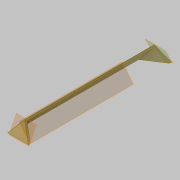
# Autodesk Inventor part: ESTAMP Post 6832 Gold L=149; BC=128
Saved by Autodesk Inventor 2024 (Build 280153000, 153)
## iProperties
Created: 2023-02-20
Part Number: ESTAMP Post 6832 Gold L=149; BC=128
Material: Zinc
Document SubType Name: Modeling
Designer: sauliusd
Density: 7 g/cm^3
Appearance: Gold - Metal
Description: ESTAMP Handle Post 683
Appearance: Chrome - Polished Black
Author: sauliusd
Autodesk Inventor part; units mm, degrees
ref_plane "YZ Plane" through (0, 0, 0) normal (1, 0, 0) x (0, 1, 0)
ref_plane "XZ Plane" through (0, 0, 0) normal (0, 1, 0) x (-1, 0, 0)
ref_plane "XY Plane" through (0, 0, 0) normal (0, 0, 1) x (1, 0, 0)
sketch "Sketch1" plane through (0, 0, 0) normal (0, 0, 1) x (1, 0, 0)
  line L0 (-106.5, -15.5) -> (106.5, -15.5)
  line L1 (106.5, -15.5) -> (106.5, 15.5)
  line L2 (106.5, 15.5) -> (-106.5, 15.5)
  line L3 (-106.5, 15.5) -> (-106.5, -15.5)
  line L4 (-106.5, -15.5) -> (106.5, 15.5) construction
  line L5 (106.5, -15.5) -> (-106.5, 15.5) construction
  point P0 (0, 0)
  dimension "L" = 213
  dimension "d1" = 31
  constraints: 12 end point, 2 midpoint, 2 parallel, 1 horizontal, 1 perpendicular
  measures "L" distance of L2.end L1.end
  measures "d1" distance of L1.end L0.end
extrude "Extrusion1" add sketch "Sketch1" along normal blind 20
sketch "Sketch2" plane through (106.5, -15.5, 0) normal (1, 0, 0) x (0, 0, -1)
  line L0 (0, 0) -> (-20, 0) projected
  line L1 (0, 0) -> (-20, 15.5)
  line L2 (-20, 0) -> (-20, 31) projected
  point P0 (0, 15.5)
  constraints: 2 end point, 1 midpoint
extrude "Extrusion2" cut sketch "Sketch2" against normal through all
mirror "Mirror1" about plane through (0, 0, 0) normal (0, 1, 0) of "Extrusion2"
sketch "Sketch3" plane through (0, 0, 0) normal (0, 1, 0) x (-1, 0, 0)
  line L0 (106.5, 0) -> (-106.5, 0) projected
  line L1 (-106.5, 0) -> (-96.5, 20)
  line L2 (106.5, 20) -> (-106.5, 20) projected
  line L3 (-106.5, 0) -> (-106.5, 20) projected
  point P0 (0, 0)
  dimension "d6" = 10
  constraints: 2 end point, 1 point on line
  measures "d6" distance from line of L3 L1.end
extrude "Extrusion3" cut sketch "Sketch3" along normal through all both and the other way through all
mirror "Mirror2" about plane through (0, 0, 0) normal (1, 0, 0) of "Extrusion3"
shell "Shell1" thickness 2.5 removed faces 2 at (-32.1667, -10.3333, 6.6667) at (35.5, -5.1667, 0)
sketch "Sketch4" plane through (0, 0, 0) normal (0, 0, 1) x (1, 0, 0)
  line L0 (-106.5, -15.5) -> (-103.7049, -15.5) projected
  line L1 (-103.7049, -15.5) -> (-85.5, 12.3371)
  line L2 (103.7049, 12.3371) -> (-103.7049, 12.3371) projected
  line L3 (-106.5, 15.5) -> (-106.5, -15.5) projected
  line L4 (-103.7049, 12.3371) -> (-103.7049, -15.5) projected
  point P0 (0, 0)
  dimension "d10" = 21
  constraints: 2 end point, 1 point on line
  measures "d10" distance from line of L3 L1.end
extrude "Extrusion4" add sketch "Sketch4" along normal up to surface surface through (106.5, -1.976, 18.4686) normal (0, -0.7904151, -0.6125717)
ref_plane "Work Plane1" through (-106.5, -15.5, 0) normal (-0.8944272, 0, 0.4472136) x (0.4472136, 0, 0.8944272)
split "Split1" plane through (-106.5, -15.5, 0) removes the side toward (-0.8944272, 0, 0.4472136)
ref_plane "Work Plane2" through (-96.5, 0, 20) normal (0, -0.7904151, 0.6125717) x (1, 0, 0)
split "Split2" plane through (-96.5, 0, 20) removes the side toward (0, -0.7904151, 0.6125717)
mirror "Mirror3" about plane through (0, 0, 0) normal (1, 0, 0) of "Extrusion4", "Split1", "Split2"
fillet "Fillet1" radius 0.3 4 edges at (-101.5, 7.75, 10) (-101.5, -7.75, 10) (101.5, 7.75, 10) (101.5, -7.75, 10)
fillet "Fillet2" radius 0.3 3 edges at (96.4817, 0, 19.9011) (-96.4817, 0, 19.9011) (0, 0, 20)
sketch "Sketch5" plane through (0, 0, 0) normal (0, 0, -1) x (-1, 0, 0)
  line L0 (-96, 3.5) -> (96, 3.5)
  line L1 (-106.2565, 15.5) -> (106.2565, 15.5) projected
  point P0 (0, 0)
  point P1 (0, 3.5)
  dimension "d17" = 12
  dimension "BC" = 192
  constraints: 2 end point, 1 horizontal, 1 midpoint, 1 vertical alignment
  measures "d17" distance between parallel lines of L1 L0
  measures "BC" distance of L0.start L0.end
hole "Hole1" at (96, 3.5, 0) at (-96, 3.5, 0) direction (0, 0, 1) diameter 3.242 depth 11 tip angle 118 thread size "M4x0.7" class "6H" standard "ISO Metric profile"
chamfer "Chamfer1" distance 0.2 angle 45 2 edges at (96, 1.879, 0) (-96, 1.879, 0)
ref_plane "Work Plane3" through (106.5, -15.5, 0) normal (-0.8944272, 0, -0.4472136) x (-0.4472136, 0, 0.8944272)
body "Solid1"
